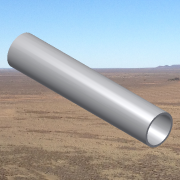
# Autodesk Inventor part: 2h3cond
Saved by Autodesk Inventor 2013 SP2 (Build 170200200, 200)
## iProperties
Company: HERA Project
Created: 2013-05-21
Part Number: 2h3cond
Material: PVC-Piping
Document SubType Name: Modeling
Designer: David DeBoer
Density: 1.4 g/cm^3
Description: Hub signal/power conduit
Mass: 295.821 g
Surface Area: 1094.25 cm^2
Volume: 211.301 cm^3
Author: David DeBoer
Autodesk Inventor part; units mm, degrees
ref_plane "YZ Plane" through (0, 0, 0) normal (1, 0, 0) x (0, 1, 0)
ref_plane "XZ Plane" through (0, 0, 0) normal (0, 1, 0) x (-1, 0, 0)
ref_plane "XY Plane" through (0, 0, 0) normal (0, 0, 1) x (1, 0, 0)
sketch "Sketch3" plane through (0, 0, 0) normal (1, 0, 0) x (0, 1, 0)
  circle A0 centre (0, 0) radius 30.1625
  circle A1 centre (0, 0) radius 26.2509
  dimension "d4" = 60.325
  dimension "d5" = 3.9116
  constraints: 2 centre point, 1 coincident
  measures "d4" diameter of A0
  measures "d5" radial gap between concentric circles of A1 A0
extrude "Extrusion2" add sketch "Sketch3" along normal blind 304.8
body "Solid2"
